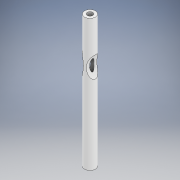
# Autodesk Inventor part: Fillament Guide
Saved by Autodesk Inventor 2020.2 (Build 242310000, 310)
## iProperties
Created: 2020-03-03
Part Number: Fillament Guide
Material: Polypropylene
Document SubType Name: Modeling
Designer: Richard Hall
Density: 0.899 g/cm^3
Appearance: Smooth - White
Author: Richard Hall
Title: Fillament Guide
Autodesk Inventor part; units mm, degrees
ref_plane "YZ Plane" through (0, 0, 0) normal (1, 0, 0) x (0, 1, 0)
ref_plane "XZ Plane" through (0, 0, 0) normal (0, 1, 0) x (-1, 0, 0)
ref_plane "XY Plane" through (0, 0, 0) normal (0, 0, 1) x (1, 0, 0)
sketch "Sketch1" plane through (0, 0, 0) normal (0, 1, 0) x (-1, 0, 0)
  circle A0 centre (0, 0) radius 2
  circle A1 centre (0, 0) radius 1
  dimension "d0" = 4
  dimension "d3" = 1
  constraints: 2 centre point, 1 coincident
  measures "d0" diameter of A0
  measures "d3" radial gap between concentric circles of A1 A0
extrude "Extrusion1" add sketch "Sketch1" along normal mid plane 48.3
sketch "Sketch2" plane through (0, 0, 0) normal (0, 0, 1) x (1, 0, 0)
  circle A0 centre (6.1, 8.35) radius 5.5 construction
  line L0 (2, 24.15) -> (-2, 24.15) projected
  circle A1 centre (-9, 8.35) radius 8.5
  line L1 (-0.875, -5) -> (0.875, -5)
  line L2 (0.875, -5) -> (0.875, 5)
  line L3 (0.875, 5) -> (-0.875, 5)
  line L4 (-0.875, 5) -> (-0.875, -5)
  line L5 (-0.875, -5) -> (0.875, 5)
  line L6 (0.875, -5) -> (-0.875, 5)
  circle A2 centre (6.6, 8.35) radius 6
  line L7 (1, 24.15) -> (1, -24.15) projected
  line L8 (-2, -24.15) -> (2, -24.15) projected
  point P0 (0, 0)
  point P1 (0.875, 4.8043)
  point P2 (0.875, 4.7957)
  dimension "d6" = 11
  dimension "d8" = 17
  dimension "d12" = 1.75
  dimension "d13" = 10
  dimension "d18" = 12
  dimension "d20" = 1.5
  dimension "d21" = 1.1
  dimension "d25" = 9
  dimension "d26" = 15.8
  constraints: 12 end point, 3 centre point, 3 horizontal alignment, 2 midpoint, 2 parallel, 1 horizontal, 1 perpendicular, 1 tangent
  measures "d6" diameter of A0
  measures "d8" diameter of A1
  measures "d12" distance of L3.end L2.end
  measures "d13" distance of L2.end L1.end
  measures "d18" diameter of A2
  measures "d20" distance edge to line of A1 L7
  measures "d25" horizontal distance of A1.centre point (0, 0)
  measures "d26" vertical distance of L7.start A2.centre
extrude "Extrusion2" cut sketch "Sketch2" along normal mid plane 10 contours A1 | A2 L7 | L7 A2
body "Solid1"
